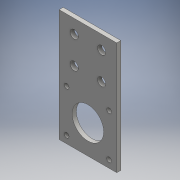
# Autodesk Inventor part: 电机座3
Saved by Autodesk Inventor 2016 (Build 200138000, 138)
## iProperties
Created: 2019-04-02
Part Number: 电机座3
Material: 常规
Document SubType Name: Modeling
Designer: oldboy
Density: 1 g/cm^3
Appearance: 默认
Author: oldboy
Autodesk Inventor part; units mm, degrees
ref_plane "YZ Plane" through (0, 0, 0) normal (1, 0, 0) x (0, 1, 0)
ref_plane "XZ Plane" through (0, 0, 0) normal (0, 1, 0) x (-1, 0, 0)
ref_plane "XY Plane" through (0, 0, 0) normal (0, 0, 1) x (1, 0, 0)
sketch "草图2" plane through (0, 0, 0) normal (0, 1, 0) x (-1, 0, 0)
  line L0 (-21, 21) -> (21, 21)
  line L1 (21, 21) -> (21, -21)
  line L2 (21, -21) -> (-21, -21)
  line L3 (-21, -21) -> (-21, 21)
  line L4 (-21, 21) -> (21, -21) construction
  line L5 (21, 21) -> (-21, -21) construction
  point P0 (0, 0)
  dimension "d3" = 42
  dimension "d4" = 42
  constraints: 12 end point, 2 midpoint, 2 parallel, 1 horizontal, 1 perpendicular
  measures "d3" distance between parallel lines of L3 L1
  measures "d4" distance between parallel lines of L2 L0
extrude "拉伸2" add sketch "草图2" along normal blind 3
sketch "草图7" plane through (0, 0, 0) normal (0, -1, 0) x (1, 0, 0)
  circle A0 centre (0, 0) radius 11.5
  circle A1 centre (-15.5, 15.5) radius 1.75
  circle A2 centre (-15.5, -15.5) radius 1.75
  circle A3 centre (15.5, -15.5) radius 1.75
  circle A4 centre (15.5, 15.5) radius 1.75
  dimension "d17" = 23
  dimension "d18" = 3.5
  dimension "d19" = 15.5
  dimension "d20" = 15.5
  dimension "d21" = 15.5
  dimension "d22" = 15.5
  constraints: 5 centre point, 3 equal radius, 2 horizontal alignment, 2 vertical alignment, 1 coincident
  measures "d17" diameter of A0
  measures "d18" diameter of A2
  measures "d19" horizontal distance of point (0, 0) A2.centre
  measures "d20" horizontal distance of point (0, 0) A2.centre
  measures "d21" horizontal distance of point (0, 0) A1.centre
  measures "d22" horizontal distance of point (0, 0) A3.centre
extrude "拉伸6" cut sketch "草图7" against normal blind 3
sketch "草图14" plane through (-21, 0, 21) normal (0, 0, 1) x (1, 0, 0)
  line L0 (42, 0) -> (0, 0) projected
  line L1 (42, 0) -> (42, 3) projected
  line L2 (0, 3) -> (42, 3) projected
  line L3 (0, 0) -> (0, 3) projected
  point P0 (21, 0)
extrude "拉伸13" add sketch "草图14" along normal blind 40
sketch "草图15" plane through (0, 0, 0) normal (0, -1, 0) x (1, 0, 0)
  line L0 (0, 77.4) -> (0, -37.4) construction
  circle A0 centre (10, 51) radius 3
  line L1 (-21, 61) -> (21, 61) projected
  circle A1 centre (10, 31) radius 3
  circle A2 centre (-10, 51) radius 3
  circle A3 centre (-10, 31) radius 3
  point P0 (0, 0)
  dimension "d51" = 6
  dimension "d52" = 10
  dimension "d53" = 10
  dimension "d54" = 6
  dimension "d55" = 20
  constraints: 4 centre point, 2 symmetric about line, 1 vertical alignment, 2 other
  measures "d51" diameter of A0
  measures "d52" distance from line of L0 A0.centre
  measures "d53" distance from line of L1 A0.centre
  measures "d54" diameter of A1
  measures "d55" distance of A0.centre A1.centre
extrude "拉伸14" cut sketch "草图15" against normal blind 40
